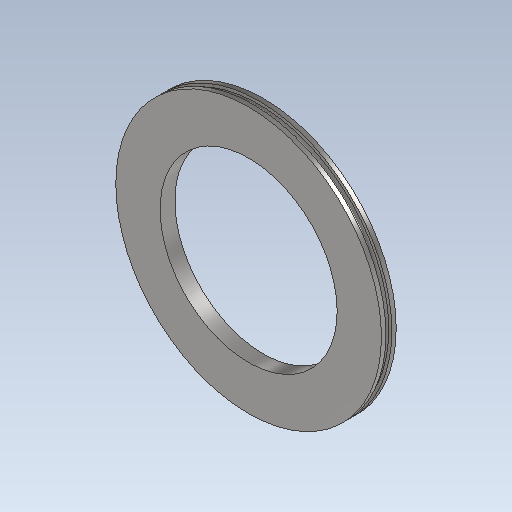
# Autodesk Inventor part: Кольцо сальника_CPY
Saved by Autodesk Inventor 2021 (Build 250183000, 183)
## iProperties
Created: 2020-11-05
Part Number: Кольцо сальника_CPY
Material: Сталь, легированная
Document SubType Name: Modeling
Designer: Тимоха
Mass: 128.953 g
Surface Area: 102.745 cm^2
Volume: 16.6822 cm^3
Density: 7.73 g/cm^3
Appearance: С умеренной полировкой
Author: Тимоха
Autodesk Inventor part; units mm, degrees
ref_plane "YZ Plane" through (0, 0, 0) normal (1, 0, 0) x (0, 1, 0)
ref_plane "XZ Plane" through (0, 0, 0) normal (0, 1, 0) x (-1, 0, 0)
ref_plane "XY Plane" through (0, 0, 0) normal (0, 0, 1) x (1, 0, 0)
sketch "Эскиз1" plane through (0, 0, 0) normal (0, 0, 1) x (1, 0, 0)
  circle A0 centre (0, 0) radius 30
  circle A1 centre (0, 0) radius 45
  dimension "d0" = 60
  dimension "d1" = 90
  constraints: 2 centre point, 2 coincident
  measures "d0" diameter of A0
  measures "d1" diameter of A1
extrude "Выдавливание1" add sketch "Эскиз1" along normal blind 5
sketch "Эскиз2" plane through (0, 0, 0) normal (1, 0, 0) x (0, 1, 0)
  line L0 (-45, 0) -> (-45, 5) projected
  line L1 (0, -0.8) -> (0, 4.8) projected
  line L2 (-45, 0) -> (-45, 5) projected
  line L3 (-45, 2.5) -> (-44, 2.5)
  circle A0 centre (-44, 2.5) radius 1
  line L4 (-44, 3.5) -> (-45, 3.5)
  line L5 (-44, 1.5) -> (-45, 1.5)
  line L6 (-45, 0) -> (-45, 5) projected
  point P0 (0, 0)
  dimension "d6" = 1
  dimension "d7" = 2
  constraints: 6 end point, 2 perpendicular, 2 point on circle, 2 point on line, 2 tangent, 1 centre point, 1 coincident, 1 horizontal, 1 midpoint
  measures "d6" distance of L3.start L3.end
  measures "d7" diameter of A0
revolve "Вращение1" cut sketch "Эскиз2" angle 360 about axis through (0, 0, -10) along (0, 0, 1)
